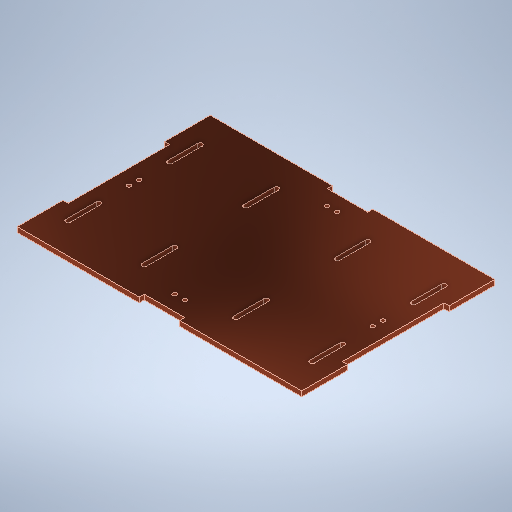
# Autodesk Inventor part: base_2
Saved by Autodesk Inventor 2025.3 (Build 293356030, 356C)
## iProperties
Created: 2026-06-26
Part Number: base_2
Material: Generic
Document SubType Name: Modeling
Designer: user
Density: 1 g/cm^3
Appearance: Copper - Polished
Author: user
Autodesk Inventor part; units mm, degrees
ref_plane "YZ Plane" through (0, 0, 0) normal (1, 0, 0) x (0, 1, 0)
ref_plane "XZ Plane" through (0, 0, 0) normal (0, 1, 0) x (-1, 0, 0)
ref_plane "XY Plane" through (0, 0, 0) normal (0, 0, 1) x (1, 0, 0)
sketch "Sketch1" plane through (0, 0, 0) normal (0, 1, 0) x (-1, 0, 0)
  line L0 (0, 0) -> (-280, 0)
  line L1 (-280, 0) -> (-280, -190)
  line L2 (-280, -190) -> (0, -190)
  line L3 (5, -95) -> (-280, -95) construction
  line L4 (-140, 0) -> (-140, -190) construction
  line L5 (-57.5, 0) -> (-57.5, -190) construction
  line L6 (-203, 0) -> (-203, -190) construction
  line L7 (-20, -160) -> (-20, -130) construction
  line L8 (-20, -160) -> (-20, -130) construction
  line L9 (-17.75, -160) -> (-17.75, -130)
  line L10 (-22.25, -130) -> (-22.25, -160)
  arc A0 (-22.25, -160) -> (-17.75, -160) centre (-20, -160) ccw
  arc A1 (-17.75, -130) -> (-22.25, -130) centre (-20, -130) ccw
  line L11 (-95, -160) -> (-95, -130) construction
  line L12 (-95, -160) -> (-95, -130) construction
  line L13 (-97.25, -160) -> (-97.25, -130)
  line L14 (-92.75, -130) -> (-92.75, -160)
  arc A2 (-97.25, -160) -> (-92.75, -160) centre (-95, -160) ccw
  arc A3 (-92.75, -130) -> (-97.25, -130) centre (-95, -130) ccw
  line L15 (-160, -190) -> (-120, -190)
  line L16 (-120, -190) -> (-120, -185)
  line L17 (-120, -185) -> (-160, -185)
  line L18 (-160, -185) -> (-160, -190)
  line L19 (-260, -160) -> (-260, -130) construction
  line L20 (-260, -160) -> (-260, -130) construction
  line L21 (-262.25, -160) -> (-262.25, -130)
  line L22 (-257.75, -130) -> (-257.75, -160)
  arc A4 (-262.25, -160) -> (-257.75, -160) centre (-260, -160) ccw
  arc A5 (-257.75, -130) -> (-262.25, -130) centre (-260, -130) ccw
  line L23 (-187.25, -130) -> (-187.25, -160)
  line L24 (-185, -160) -> (-185, -130) construction
  line L25 (-182.75, -160) -> (-182.75, -130)
  arc A6 (-187.25, -160) -> (-182.75, -160) centre (-185, -160) ccw
  line L26 (-185, -160) -> (-185, -130) construction
  arc A7 (-182.75, -130) -> (-187.25, -130) centre (-185, -130) ccw
  line L27 (-140, -190) -> (-140, 0) construction
  line L28 (-20, -30) -> (-20, -60) construction
  line L29 (-20, -30) -> (-20, -60) construction
  line L30 (-17.75, -30) -> (-17.75, -60)
  line L31 (-22.25, -60) -> (-22.25, -30)
  arc A8 (-17.75, -30) -> (-22.25, -30) centre (-20, -30) ccw
  arc A9 (-22.25, -60) -> (-17.75, -60) centre (-20, -60) ccw
  line L32 (-92.75, -60) -> (-92.75, -30)
  line L33 (-95, -30) -> (-95, -60) construction
  line L34 (-97.25, -30) -> (-97.25, -60)
  arc A10 (-92.75, -30) -> (-97.25, -30) centre (-95, -30) ccw
  line L35 (-95, -30) -> (-95, -60) construction
  arc A11 (-97.25, -60) -> (-92.75, -60) centre (-95, -60) ccw
  line L36 (-160, 0) -> (-120, 0)
  line L37 (-120, 0) -> (-120, -5)
  line L38 (-120, -5) -> (-160, -5)
  line L39 (-160, -5) -> (-160, 0)
  arc A12 (-257.75, -30) -> (-262.25, -30) centre (-260, -30) ccw
  line L40 (-257.75, -60) -> (-257.75, -30)
  line L41 (-260, -30) -> (-260, -60) construction
  line L42 (-260, -30) -> (-260, -60) construction
  arc A13 (-262.25, -60) -> (-257.75, -60) centre (-260, -60) ccw
  line L43 (-262.25, -30) -> (-262.25, -60)
  line L44 (-187.25, -60) -> (-187.25, -30)
  line L45 (-185, -30) -> (-185, -60) construction
  line L46 (-185, -30) -> (-185, -60) construction
  arc A14 (-187.25, -60) -> (-182.75, -60) centre (-185, -60) ccw
  line L47 (-182.75, -30) -> (-182.75, -60)
  arc A15 (-182.75, -30) -> (-187.25, -30) centre (-185, -30) ccw
  line L48 (-280, -42.5) -> (-280, -92.5)
  line L49 (-280, -92.5) -> (-280, -145)
  line L50 (-280, -145) -> (-275, -145)
  line L51 (-275, -145) -> (-275, -45)
  line L52 (-275, -45) -> (-280, -45)
  line L53 (-280, -45) -> (-280, -42.5)
  line L54 (5, -45) -> (-5, -45)
  line L55 (-5, -45) -> (-5, -145)
  line L56 (-5, -145) -> (5, -145)
  line L57 (0, -190) -> (0, 0)
  point P0 (-20, -145)
  point P1 (-95, -145)
  point P2 (-260, -145)
  point P3 (-185, -145)
  point P4 (-20, -45)
  point P5 (-95, -45)
  point P6 (-260, -45)
  point P7 (-185, -45)
  point P8 (-95, -145)
  point P9 (-20, -145)
  point P10 (-280, -45)
  point P11 (-160, -190)
  point P12 (-120, -190)
  point P13 (-120, 0)
  point P14 (-160, 0)
  point P15 (-260, -145)
  point P16 (0, -45)
  point P17 (0, -145)
  dimension "d2" = 30
  dimension "d4" = 30
  dimension "d6" = 2.25
  dimension "d9" = 40
  dimension "d13" = 0
  dimension "d14" = 5
  dimension "d16" = 20
  dimension "d21" = 10
  dimension "d22" = 5
  dimension "d26" = 50
  dimension "d27" = 50
  dimension "d28" = 0
  dimension "d30" = 190
  dimension "d32" = 75
  dimension "d34" = 100
  dimension "d36" = 50
  dimension "d56" = 20
  dimension "d57" = 280
  constraints: 132 end point, 55 symmetric about line, 32 point on circle, 16 centre point, 7 midpoint, 6 equal length, 6 perpendicular, 5 point on line, 4 tangent, 3 horizontal, 1 vertical, 14 other
  measures "d2" distance of L7.start L7.end
  measures "d4" distance from line of L2 L7.start
  measures "d6" radius of A0
  measures "d9" distance of L17.end L16.end
  measures "d13" distance between parallel lines of L2 L15
  measures "d14" distance between parallel lines of L17 L15
  measures "d16" distance between parallel lines of L4 L18
  measures "d21" distance of L56.end L55.end
  measures "d22" distance between parallel lines of L49 L51
  measures "d26" distance between parallel lines of L3 L52
  measures "d27" distance between parallel lines of L3 L50
  measures "d28" distance between parallel lines of L1 L48
  measures "d30" distance between parallel lines of L0 L2
  measures "d32" distance of point (-95, -145) point (-20, -145)
  measures "d34" distance between parallel lines of L56 L54
  measures "d36" distance between parallel lines of L54 L3
  measures "d56" distance from line of L1 point (-260, -145)
  measures "d57" distance between parallel lines of L1 L57
extrude "Extrusion1" add sketch "Sketch1" along normal blind 5 contours L57 L54 L55 L56 L2 L16 L17 L18 L1 L50 L51 L52 L0 L39 L38 L37
sketch "Sketch2" plane through (0, 5, 0) normal (0, 1, 0) x (1, 0, 0)
  line L0 (160, 185) -> (120, 185) projected
  line L1 (120, 185) -> (120, 190) projected
  line L2 (160, 5) -> (160, 0) projected
  line L3 (160, 0) -> (280, 0) projected
  line L4 (5, 145) -> (5, 45) projected
  point P0 (0, 0)
  point P1 (135, 20)
  point P2 (145, 20)
  point P3 (135, 170)
  point P4 (145, 170)
  point P5 (20, 90)
  point P6 (20, 100)
  dimension "d44" = 10
  dimension "d45" = 10
  dimension "d46" = 10
  dimension "d47" = 15
  dimension "d48" = 15
  dimension "d49" = 15
  dimension "d50" = 15
  dimension "d51" = 20
  dimension "d52" = 20
  dimension "d53" = 15
  dimension "d54" = 15
  dimension "d55" = 45
  measures "d44" distance of point (135, 170) point (145, 170)
  measures "d45" distance of point (135, 20) point (145, 20)
  measures "d46" distance of point (20, 90) point (20, 100)
  measures "d47" distance from line of L0 point (135, 170)
  measures "d48" distance from line of L0 point (145, 170)
  measures "d49" distance from line of L1 point (135, 170)
  measures "d50" distance from line of L2 point (145, 20)
  measures "d51" distance from line of L3 point (145, 20)
  measures "d52" distance from line of L3 point (135, 20)
  measures "d53" distance from line of L4 point (20, 100)
  measures "d54" distance from line of L4 point (20, 90)
  measures "d55" vertical distance of L4.start point (20, 100)
hole "Hole1" at (135, 5, -20) at (145, 5, -20) at (135, 5, -170) at (145, 5, -170) at (20, 5, -90) at (20, 5, -100) direction (0, -1, 0) diameter 4 end through all
sketch "Sketch3" plane through (0, 5, 0) normal (0, 1, 0) x (1, 0, 0)
  line L0 (275, 145) -> (280, 145) projected
  line L1 (275, 45) -> (275, 145) projected
  point P0 (0, 0)
  point P1 (260, 90)
  point P2 (260, 100)
  dimension "d65" = 45
  dimension "d66" = 10
  dimension "d67" = 15
  dimension "d68" = 15
  measures "d65" distance from line of L0 point (260, 100)
  measures "d66" distance of point (260, 90) point (260, 100)
  measures "d67" distance from line of L1 point (260, 100)
  measures "d68" distance from line of L1 point (260, 90)
hole "Hole2" at (260, 5, -90) at (260, 5, -100) direction (0, -1, 0) diameter 4 end through all
body "Solid1"
